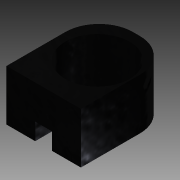
# Autodesk Inventor part: supporto_manicotto_X
Saved by Autodesk Inventor 2014 SP1 (Build 180222100, 222)
## iProperties
Created: 2015-04-08
Part Number: supporto_manicotto_X
Material: Generic
Document SubType Name: Modeling
Designer: Giorgio Nuzzo
Density: 1 g/cm^3
Appearance: Fine Textured - Black
d0: 27,390 mm
d1: 22,000 mm
d2: 10,000 mm
d3: 15,000 mm
d4: 11,500 mm
d5: 15,000 mm
d6: 0,00 deg
d7: 10,000 mm
d8: 5,000 mm
d9: 5,000 mm
d10: 0,00 deg
d11: 11,000 mm
Author: Giorgio Nuzzo
Autodesk Inventor part; units mm, degrees
ref_plane "YZ Plane" through (0, 0, 0) normal (1, 0, 0) x (0, 1, 0)
ref_plane "XZ Plane" through (0, 0, 0) normal (0, 1, 0) x (-1, 0, 0)
ref_plane "XY Plane" through (0, 0, 0) normal (0, 0, 1) x (1, 0, 0)
sketch "Sketch1" plane through (0, 0, 0) normal (0, 0, 1) x (1, 0, 0)
  line L0 (11, -13.695) -> (-11, -13.695)
  line L1 (-11, -13.695) -> (-11, 3.695)
  line L2 (-1, 13.695) -> (1, 13.695)
  line L3 (11, 3.695) -> (11, -13.695)
  line L4 (11, -13.695) -> (-11, 13.695) construction
  line L5 (-11, -13.695) -> (11, 13.695) construction
  arc A0 (-1, 13.695) -> (-11, 3.695) centre (-1, 3.695) ccw
  arc A1 (11, 3.695) -> (1, 13.695) centre (1, 3.695) ccw
  circle A2 centre (0, 2.195) radius 7.5
  point P0 (0, 0)
  dimension "d0" = 27.39
  dimension "d1" = 22
  dimension "d2" = 10
  dimension "d3" = 15
  dimension "d4" = 11.5
  dimension "d11" = 11
  constraints: 12 end point, 4 point on circle, 4 point on line, 4 tangent, 3 centre point, 2 midpoint, 2 parallel, 1 equal radius, 1 horizontal, 1 perpendicular
  measures "d0" distance of L0.end L4.end
  measures "d1" distance of L4.end L5.end
  measures "d2" radius of A0
  measures "d3" diameter of A2
  measures "d4" distance from line of L2 A2.centre
  measures "d11" distance from line of L1 A2.centre
extrude "Extrusion1" add sketch "Sketch1" along normal blind 15
sketch "Sketch2" plane through (0, 0, 0) normal (0, 0, -1) x (-1, 0, 0)
  line L0 (-11, -13.695) -> (11, -13.695) projected
  line L1 (-2.5, -13.695) -> (2.5, -13.695)
  line L2 (2.5, -13.695) -> (2.5, -3.695)
  line L3 (2.5, -3.695) -> (-2.5, -3.695)
  line L4 (-2.5, -3.695) -> (-2.5, -13.695)
  line L5 (0, -19.173) -> (0, 19.173) construction
  point P0 (0, 0)
  dimension "d7" = 10
  dimension "d8" = 5
  constraints: 8 end point, 2 parallel, 1 horizontal, 1 perpendicular, 1 point on line, 1 other
  measures "d7" distance of L1.end L2.end
  measures "d8" distance between parallel lines of L4 L2
extrude "Extrusion2" cut sketch "Sketch2" against normal blind 5
equation "\"d11\" = 0.5 * d1"
body "Solid1"
